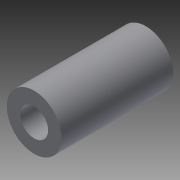
# Autodesk Inventor part: standoff(so)
Saved by Autodesk Inventor 2015 SP1 (Build 190203100, 203)
## iProperties
Created: 2015-10-03
Part Number: standoff(so)
Material: Generic
Document SubType Name: Modeling
Designer: elilitwack
Density: 1 g/cm^3
Appearance: Default
Author: elilitwack
Autodesk Inventor part; units mm, degrees
ref_plane "YZ Plane" through (0, 0, 0) normal (1, 0, 0) x (0, 1, 0)
ref_plane "XZ Plane" through (0, 0, 0) normal (0, 1, 0) x (-1, 0, 0)
ref_plane "XY Plane" through (0, 0, 0) normal (0, 0, 1) x (1, 0, 0)
sketch "profile_sketch" plane through (0, 0, 0) normal (0, 0, 1) x (1, 0, 0)
  circle A0 centre (0, 0) radius 3.175
  circle A1 centre (0, 0) radius 6.223
  dimension "d0" = 6.35
  dimension "d1" = 3.048
  constraints: 2 centre point, 2 coincident
  measures "d0" diameter of A0
  measures "d1" radial gap between concentric circles of A0 A1
extrude "profile_extrusion" add sketch "profile_sketch" along normal blind 25.4
equation "\"d0\" = so_inner_diameter"
equation "\"d1\" = so_wall_thickness"
equation "\"d2\" = so_length"
equation "\"so_inner_diameter\" = 6.35"
equation "\"so_wall_thickness\" = 3.048"
equation "\"so_length\" = 25.4"
body "Solid1"
